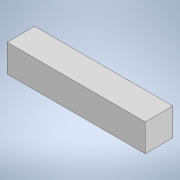
# Autodesk Inventor part: Part7
Saved by Autodesk Inventor 2022 (Build 260153070, 153G)
## iProperties
Created: 2021-07-07
Part Number: Part7
Material: Generic
Document SubType Name: Modeling
Designer: sachin
Density: 1 g/cm^3
Appearance: Default
Author: sachin
Autodesk Inventor part; units mm, degrees
ref_plane "YZ Plane" through (0, 0, 0) normal (1, 0, 0) x (0, 1, 0)
ref_plane "XZ Plane" through (0, 0, 0) normal (0, 1, 0) x (-1, 0, 0)
ref_plane "XY Plane" through (0, 0, 0) normal (0, 0, 1) x (1, 0, 0)
sketch "Sketch1" plane through (0, 0, 0) normal (0, 0, 1) x (1, 0, 0)
  line L0 (-124.7074, 87.4321) -> (129.2926, 87.4321)
  line L1 (129.2926, 87.4321) -> (129.2926, 36.6321)
  line L2 (129.2926, 36.6321) -> (-124.7074, 36.6321)
  line L3 (-124.7074, 36.6321) -> (-124.7074, 87.4321)
  point P0 (0, 0)
  dimension "d0" = 254
  dimension "d1" = 50.8
  constraints: 8 end point, 2 parallel, 1 horizontal, 1 perpendicular
  measures "d0" distance of L0.start L0.end
  measures "d1" distance of L0.end L1.end
extrude "Extrusion1" add sketch "Sketch1" along normal blind 50.8
body "Solid1"
